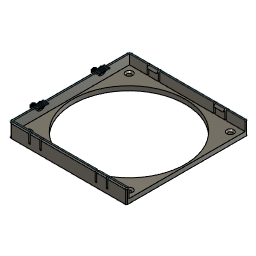
Arctic_Freezer_4U_SP3_120mm_fan_adapter v1 (Autodesk Fusion 360 design; units mm, degrees)
Autodesk Fusion 360 part; units mm, degrees
sketch "Sketch1" plane through (0, 0, 0) normal (0, 1, 0) x (1, 0, 0)
  line L0 (60, 60.25) -> (-60, 60.25)
  line L1 (-60, 60.25) -> (-60, -60.25)
  line L2 (-60, -60.25) -> (60, -60.25)
  line L3 (60, -60.25) -> (60, 60.25)
  line L4 (60, 60.25) -> (-60, -60.25) construction
  line L5 (-60, 60.25) -> (60, -60.25) construction
  dimension "d1" = 120
  dimension "d2" = 120.5
  constraint horizontal L0
  constraint perpendicular L0 L1
  constraint parallel L0 L2
  constraint parallel L1 L3
  constraint coincident L4 origin
  constraint coincident L5 origin
  measures "d1" distance of L1.end L2.end
  measures "d2" distance of L0.end L1.end
extrude "Extrude1" add sketch "Sketch1" along normal blind 4.5
sketch "Sketch2" plane through (0, 4.5, 0) normal (0, 1, 0) x (-1, 0, 0)
  line L0 (-60, 60.25) -> (-60, -60.25)
  line L1 (-60, -60.25) -> (60, -60.25)
  line L2 (60, -60.25) -> (60, 60.25)
  line L3 (60, 60.25) -> (-60, 60.25)
  line L4 (-52.5, -52.5) -> (52.5, -52.5) construction
  line L5 (52.5, -52.5) -> (52.5, 52.5) construction
  line L6 (52.5, 52.5) -> (-52.5, 52.5) construction
  line L7 (-52.5, 52.5) -> (-52.5, -52.5) construction
  line L8 (-52.5, -52.5) -> (52.5, 52.5) construction
  line L9 (52.5, -52.5) -> (-52.5, 52.5) construction
  dimension "d5" = 105
  dimension "d6" = 105
  constraint horizontal L4
  constraint perpendicular L4 L5
  constraint parallel L4 L6
  constraint parallel L5 L7
  constraint coincident L8 origin
  constraint coincident L9 origin
  measures "d5" distance of L5.end L6.end
  measures "d6" distance of L4.end L5.end
hole "Hole1" at (-52.5, 4.5, 52.5) at (-52.5, 4.5, -52.5) at (52.5, 4.5, -52.5) at (52.5, 4.5, 52.5) direction (0, -1, 0) diameter 4.4 end through all
hole "Hole2" at (-0.0995, 4.5, 0.1556) direction (0, -1, 0) diameter 117 depth 4.5 tip angle 118
extrude "Extrude2" add 1 faces at (-20, 1.5, 60.25) along direction (0, 0, 1) blind 2.5
extrude "Extrude3" add 1 faces at (-60, 1.5, 21.75) along direction (-1, 0, 0) blind 2.5
extrude "Extrude4" add 1 faces at (19.1667, 1.5, -60.25) along direction (0, 0, -1) blind 2.5
sketch "Sketch3" plane through (0, 4.5, 0) normal (0, 1, 0) x (-1, 0, 0)
  circle A0 centre (0.0995, 0.1556) radius 58.5
  circle A1 centre (-52.5, -52.5) radius 2.2
  circle A2 centre (52.5, 52.5) radius 2.2
  circle A3 centre (52.5, -52.5) radius 2.2
  circle A4 centre (-52.5, 52.5) radius 2.2
  line L0 (-60, 62.75) -> (-60, -62.75)
  line L1 (-60, -62.75) -> (62.5, -62.75)
  line L2 (62.5, -62.75) -> (62.5, 62.75)
  line L3 (62.5, 62.75) -> (-60, 62.75)
  line L4 (-60, 62.75) -> (62.5, 62.75)
  line L5 (62.5, 62.75) -> (62.5, 60.25)
  line L6 (62.5, 60.25) -> (-60, 60.25)
  line L7 (-60, 60.25) -> (-60, 62.75)
  dimension "d19" = 2.5
  constraint horizontal L4
  constraint vertical L5
  constraint horizontal L6
  constraint vertical L7
  constraint coincident L2 L5.end
  constraint coincident L0.start L3.end
  measures "d19" distance of L2.end L5.end
sketch "Sketch4" plane through (0, 4.5, 0) normal (0, 1, 0) x (-1, 0, 0)
  line L0 (-60, -62.75) -> (62.5, -62.75)
  line L1 (62.5, -62.75) -> (62.5, -60.25)
  line L2 (62.5, -60.25) -> (-60, -60.25)
  line L3 (-60, -60.25) -> (-60, -62.75)
  line L4 (62.5, 62.75) -> (62.5, -62.75)
  point P0 (-60, -62.75)
  dimension "d20" = 2.5
  constraint horizontal L0
  constraint vertical L1
  constraint horizontal L2
  constraint vertical L3
  constraint coincident L1.end L4
  constraint coincident P0 L0.start
  measures "d20" distance of L0.end L1.end
sketch "Sketch5" plane through (0, 4.5, 0) normal (0, 1, 0) x (-1, 0, 0)
  line L0 (62.5, -62.75) -> (60, -62.75)
  line L1 (60, -62.75) -> (60, 62.75)
  line L2 (60, 62.75) -> (62.5, 62.75)
  line L3 (62.5, 62.75) -> (62.5, -62.75)
  line L4 (62.5, 62.75) -> (-60, 62.75)
  point P0 (62.5, -62.75)
  dimension "d21" = 2.5
  constraint horizontal L0
  constraint vertical L1
  constraint horizontal L2
  constraint vertical L3
  constraint coincident L1.end L4
  constraint coincident P0 L0.start
  measures "d21" distance of L1.end L2.end
extrude "Extrude5" add sketch "Sketch5" sketch "Sketch4" sketch "Sketch3" along normal blind 10 of sketch 2 of sketch 3 contours L0 L2 L3 L4 L5 L6 L7
sketch "Sketch7" plane through (0, 14.5, 0) normal (0, 1, 0) x (-1, 0, 0)
  line L0 (60, 60.25) -> (60, -60.25)
  line L1 (60, -60.25) -> (-60, -60.25)
  line L2 (-60, -60.25) -> (-60, -62.75)
  line L3 (-60, -62.75) -> (62.5, -62.75)
  line L4 (62.5, -62.75) -> (62.5, 62.75)
  line L5 (62.5, 62.75) -> (-60, 62.75)
  line L6 (-60, 62.75) -> (-60, 60.25)
  line L7 (-60, 60.25) -> (60, 60.25)
  line L8 (62.5, 36.75) -> (57.5, 36.75)
  line L9 (57.5, 36.75) -> (57.5, 26.75)
  line L10 (57.5, 26.75) -> (62.5, 26.75)
  line L11 (62.5, 26.75) -> (62.5, 36.75)
  line L12 (62.5, 36.75) -> (57.5, 26.75) construction
  line L13 (57.5, 36.75) -> (62.5, 26.75) construction
  line L14 (62.5, -26.75) -> (57.5, -26.75)
  line L15 (57.5, -26.75) -> (57.5, -36.75)
  line L16 (57.5, -36.75) -> (62.5, -36.75)
  line L17 (62.5, -36.75) -> (62.5, -26.75)
  line L18 (62.5, -26.75) -> (57.5, -36.75) construction
  line L19 (57.5, -26.75) -> (62.5, -36.75) construction
  point P0 (60, 31.75)
  point P1 (60, -31.75)
  dimension "d25" = 28.5
  dimension "d26" = 10
  dimension "d43" = 28.5
  dimension "d44" = 10
  constraint horizontal L8
  constraint perpendicular L8 L9
  constraint parallel L8 L10
  constraint parallel L9 L11
  constraint coincident L4 L8.start
  constraint coincident L12 P0
  constraint coincident L13 P0
  constraint coincident L0 P0
  constraint horizontal L14
  constraint perpendicular L14 L15
  constraint parallel L14 L16
  constraint parallel L15 L17
  constraint coincident L4 L14.start
  constraint coincident L18 P1
  constraint coincident L19 P1
  constraint coincident L0 P1
  measures "d25" distance of L0.start P0
  measures "d26" distance of L8.end L9.end
  measures "d43" distance of L0.end P1
  measures "d44" distance of L14.end L15.end
extrude "Extrude8" cut sketch "Sketch7" against normal blind 5 contours L0 L4 L8 L10 L11 | L0 L4 L14 L16 L17
fillet "Fillet6" radius 5 4 edges at (-61.25, 9.5, -36.75) (-61.25, 9.5, 26.75) (-61.25, 9.5, 36.75) (-61.25, 9.5, -26.75)
fillet "Fillet8" radius 1 7 edges at (-62.5, 14.5, -49.75) (-62.5, 9.5, -31.75) (-62.5, 14.5, 0) (-62.5, 9.5, 31.75) (-62.5, 14.5, 49.75) (-1.25, 14.5, 62.75) (-1.25, 14.5, -62.75)
fillet "Fillet9" radius 3 4 edges at (-62.5, 6.75, -62.75) (-62.2071, 14.2071, -62.4571) (-62.5, 6.75, 62.75) (-62.2071, 14.2071, 62.4571)
fillet "Fillet10" radius 1 6 edges at (60, 6.75, 62.75) (60, 14.2071, 62.4571) (60, 14.5, 61) (60, 14.5, -61) (60, 14.2071, -62.4571) (60, 6.75, -62.75)
sketch "Sketch11" plane through (0, 0, -60.25) normal (0, 0, 1) x (1, 0, 0)
  arc A0 (60, 13.5) -> (59, 14.5) centre (59, 13.5) ccw
  line L0 (59, 14.5) -> (-60, 14.5)
  line L1 (-60, 14.5) -> (-60, 4.5)
  line L2 (-60, 4.5) -> (60, 4.5)
  line L3 (60, 4.5) -> (60, 13.5)
  line L4 (29, 14.5) -> (39, 14.5)
  line L5 (39, 14.5) -> (39, 12.5)
  line L6 (39, 12.5) -> (29, 12.5)
  line L7 (29, 12.5) -> (29, 14.5)
  dimension "d67" = 2
  dimension "d68" = 10
  dimension "d69" = 20
  constraint horizontal L4
  constraint vertical L5
  constraint horizontal L6
  constraint vertical L7
  constraint coincident L0 L4.start
  measures "d67" distance of L4.end L5.end
  measures "d68" distance of L5.end L6.end
  measures "d69" distance of A0.end L4.end
extrude "Extrude11" add sketch "Sketch11" along normal blind 2 contours L0 L4 L5 L6 L7
chamfer "Chamfer3" distance 2 angle 45 1 edges at (34, 14.5, -58.25)
sketch "Sketch12" plane through (0, 14.5, 0) normal (0, 1, 0) x (-1, 0, 0)
  line L0 (-39, -60.25) -> (-40.5, -60.25)
  line L1 (-40.5, -60.25) -> (-40.5, -62.75)
  line L2 (-40.5, -62.75) -> (-39, -62.75)
  line L3 (-39, -62.75) -> (-39, -60.25)
  line L4 (-60, -62.75) -> (62.5, -62.75)
  line L5 (-29, -60.25) -> (-27.5, -60.25)
  line L6 (-27.5, -60.25) -> (-27.5, -62.75)
  line L7 (-27.5, -62.75) -> (-29, -62.75)
  line L8 (-29, -62.75) -> (-29, -60.25)
  point P0 (-39, -60.25)
  point P1 (-29, -60.25)
  dimension "d73" = 1.5
  dimension "d74" = 1.5
  constraint horizontal L0
  constraint vertical L1
  constraint horizontal L2
  constraint vertical L3
  constraint coincident L1.end L4
  constraint coincident P0 L0.start
  constraint horizontal L5
  constraint vertical L6
  constraint horizontal L7
  constraint vertical L8
  constraint coincident L4 L6.end
  constraint coincident P1 L5.start
  measures "d73" distance of L1.end L2.end
  measures "d74" distance of L6.end L7.end
extrude "Extrude12" cut sketch "Sketch12" against normal blind 10
sketch "Sketch13" plane through (0, 0, -60.25) normal (0, 0, 1) x (1, 0, 0)
  line L0 (27.5, 4.5) -> (27.5, 14.5)
  line L1 (27.5, 14.5) -> (-60, 14.5)
  line L2 (-60, 14.5) -> (-60, 4.5)
  line L3 (-60, 4.5) -> (27.5, 4.5)
  line L4 (-40, 14.5) -> (-30, 14.5)
  line L5 (-30, 14.5) -> (-30, 12.5)
  line L6 (-30, 12.5) -> (-40, 12.5)
  line L7 (-40, 12.5) -> (-40, 14.5)
  dimension "d77" = 2
  dimension "d78" = 10
  dimension "d79" = 20
  constraint horizontal L4
  constraint vertical L5
  constraint horizontal L6
  constraint vertical L7
  constraint coincident L1 L4.start
  measures "d77" distance of L4.start L6.end
  measures "d78" distance of L4.start L4.end
  measures "d79" distance of L1.end L4.start
extrude "Extrude13" add sketch "Sketch13" along normal blind 2 contours L1 L4 L5 L6 L7
chamfer "Chamfer4" distance 2 angle 45 1 edges at (-35, 14.5, -58.25)
sketch "Sketch14" plane through (-1.25, 14.5, -49.75) normal (0, 1, 0) x (-1, 0, 0)
  line L0 (28.75, -10.5) -> (27.25, -10.5)
  line L1 (27.25, -10.5) -> (27.25, -13)
  line L2 (27.25, -13) -> (28.75, -13)
  line L3 (28.75, -13) -> (28.75, -10.5)
  line L4 (-61.25, -13) -> (61.25, -13)
  line L5 (38.75, -10.5) -> (40.25, -10.5)
  line L6 (40.25, -10.5) -> (40.25, -13)
  line L7 (40.25, -13) -> (38.75, -13)
  line L8 (38.75, -13) -> (38.75, -10.5)
  point P0 (28.75, -10.5)
  point P1 (38.75, -10.5)
  dimension "d83" = 1.5
  dimension "d84" = 1.5
  constraint horizontal L0
  constraint vertical L1
  constraint horizontal L2
  constraint vertical L3
  constraint coincident L1.end L4
  constraint coincident P0 L0.start
  constraint horizontal L5
  constraint vertical L6
  constraint horizontal L7
  constraint vertical L8
  constraint coincident L4 L6.end
  constraint coincident P1 L5.start
  measures "d83" distance of P0 L0.end
  measures "d84" distance of P1 L5.end
extrude "Extrude14" cut sketch "Sketch14" against normal blind 10
sketch "Sketch15" plane through (0, 0, 60.25) normal (0, 0, -1) x (-1, 0, 0)
  arc A0 (-59, 14.5) -> (-60, 13.5) centre (-59, 13.5) ccw
  line L0 (-60, 13.5) -> (-60, 4.5)
  line L1 (-60, 4.5) -> (60, 4.5)
  line L2 (60, 4.5) -> (60, 14.5)
  line L3 (60, 14.5) -> (-59, 14.5)
  line L4 (-39, 14.5) -> (-29, 14.5)
  line L5 (-29, 14.5) -> (-29, 12.5)
  line L6 (-29, 12.5) -> (-39, 12.5)
  line L7 (-39, 12.5) -> (-39, 14.5)
  dimension "d87" = 2
  dimension "d88" = 10
  dimension "d89" = 20
  constraint horizontal L4
  constraint vertical L5
  constraint horizontal L6
  constraint vertical L7
  constraint coincident L3 L4.start
  measures "d87" distance of L4.end L5.end
  measures "d88" distance of L5.end L6.end
  measures "d89" distance of A0.start L4.start
extrude "Extrude15" add sketch "Sketch15" along normal blind 2 contours L3 L4 L5 L6 L7
chamfer "Chamfer5" distance 2 angle 45 1 edges at (34, 14.5, 58.25)
sketch "Sketch17" plane through (0, 14.5, 0) normal (0, 1, 0) x (-1, 0, 0)
  line L0 (-29, 60.25) -> (-27.5, 60.25)
  line L1 (-27.5, 60.25) -> (-27.5, 62.75)
  line L2 (-27.5, 62.75) -> (-29, 62.75)
  line L3 (-29, 62.75) -> (-29, 60.25)
  line L4 (62.5, 62.75) -> (-60, 62.75)
  line L5 (-39, 60.25) -> (-40.5, 60.25)
  line L6 (-40.5, 60.25) -> (-40.5, 62.75)
  line L7 (-40.5, 62.75) -> (-39, 62.75)
  line L8 (-39, 62.75) -> (-39, 60.25)
  point P0 (-29, 60.25)
  point P1 (-39, 60.25)
  dimension "d93" = 1.5
  dimension "d94" = 1.5
  constraint horizontal L0
  constraint vertical L1
  constraint horizontal L2
  constraint vertical L3
  constraint coincident L1.end L4
  constraint coincident P0 L0.start
  constraint horizontal L5
  constraint vertical L6
  constraint horizontal L7
  constraint vertical L8
  constraint coincident L4 L6.end
  constraint coincident P1 L5.start
  measures "d93" distance of P0 L0.end
  measures "d94" distance of P1 L5.end
extrude "Extrude16" cut sketch "Sketch17" against normal blind 10
sketch "Sketch18" plane through (0, 0, 60.25) normal (0, 0, -1) x (-1, 0, 0)
  line L0 (-27.5, 14.5) -> (-27.5, 4.5)
  line L1 (-27.5, 4.5) -> (60, 4.5)
  line L2 (60, 4.5) -> (60, 14.5)
  line L3 (60, 14.5) -> (-27.5, 14.5)
  line L4 (40, 14.5) -> (30, 14.5)
  line L5 (30, 14.5) -> (30, 12.5)
  line L6 (30, 12.5) -> (40, 12.5)
  line L7 (40, 12.5) -> (40, 14.5)
  point P0 (60, 14.5)
  dimension "d97" = 10
  dimension "d98" = 2
  dimension "d99" = 20
  constraint horizontal L4
  constraint vertical L5
  constraint horizontal L6
  constraint vertical L7
  constraint coincident L3 L4.start
  measures "d97" distance of L5.end L6.end
  measures "d98" distance of L4.end L5.end
  measures "d99" distance of L4.start P0
extrude "Extrude17" add sketch "Sketch18" along normal blind 2 contours L3 L4 L5 L6 L7
chamfer "Chamfer6" distance 2 angle 45 1 edges at (-35, 14.5, 58.25)
sketch "Sketch19" plane through (0, 14.5, 0) normal (0, 1, 0) x (-1, 0, 0)
  line L0 (30, 60.25) -> (28.5, 60.25)
  line L1 (28.5, 60.25) -> (28.5, 62.75)
  line L2 (28.5, 62.75) -> (30, 62.75)
  line L3 (30, 62.75) -> (30, 60.25)
  line L4 (62.5, 62.75) -> (-60, 62.75)
  line L5 (40, 60.25) -> (41.5, 60.25)
  line L6 (41.5, 60.25) -> (41.5, 62.75)
  line L7 (41.5, 62.75) -> (40, 62.75)
  line L8 (40, 62.75) -> (40, 60.25)
  point P0 (30, 60.25)
  point P1 (40, 60.25)
  dimension "d103" = 1.5
  dimension "d104" = 1.5
  constraint horizontal L0
  constraint vertical L1
  constraint horizontal L2
  constraint vertical L3
  constraint coincident L1.end L4
  constraint coincident P0 L0.start
  constraint horizontal L5
  constraint vertical L6
  constraint horizontal L7
  constraint vertical L8
  constraint coincident L4 L6.end
  constraint coincident P1 L5.start
  measures "d103" distance of L1.end L2.end
  measures "d104" distance of P1 L5.end
extrude "Extrude18" cut sketch "Sketch19" against normal blind 10
chamfer "Chamfer7" distance 1.5 angle 45 4 edges at (-51.7044, 4.5, -54.5511) (53.2956, 4.5, -54.5511) (-51.7044, 4.5, 50.4489) (53.2956, 4.5, 50.4489)
